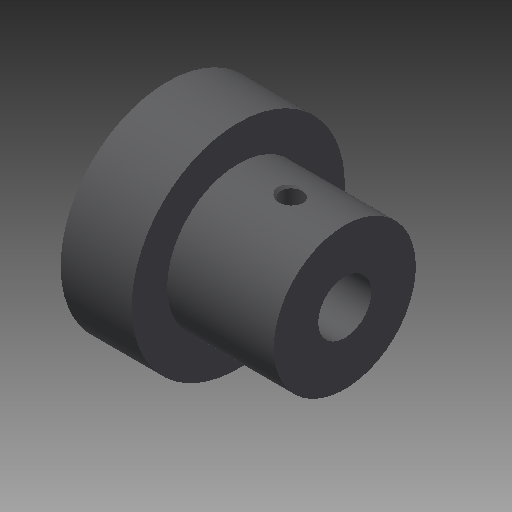
# Autodesk Inventor part: UMHSL30_c
Saved by Autodesk Inventor 2019 (Build 230136000, 136)
## iProperties
Category: PARTsolutions
Company: MISUMI
Created: 2015-12-01
Part Number: UMHSL30_c
Catalog Web Link: www.cadenas.de
Description: UMHSH, UMHS, UMHSL ,UMHAH, UMHA, UMHAL_c-Urethane Rollers with Collars
Vendor: MISUMI
Document SubType Name: Modeling
Designer: psAdmin
Manufacturer: MISUMI
Mass: 5.41814 g
Surface Area: 24.8768 cm^2
Volume: 5.41814 cm^3
Density: 1 g/cm^3
Material: Generic
Appearance: PSOLRGB-192-192-192
PSOL_IDENT_0: {$CADENAS_DATA\23d-libs\misumi\metric\53_rollers\umhsh\umhsh_c.prj},201 {VTYP=3D},{NB=UMHSL30_c},{LI
PSOL_IDENT_1: NA=UMHSL30},{NN=UMHSH, UMHS, UMHSL ,UMHAH, UMHA, UMHAL_c},{DATE=06.11.2015 05:15:16},{GEOMDATE=30.10
PSOL_IDENT_2: .2015 01:04:11},{VERSION=},{LINEID=70},{LINESUBID=-1},{WBVAR=MATC,HARD}  {NB=UMHSL30_c},{LINA=UMHSL3
PSOL_IDENT_3: 0},{KT=DUMMY},{PN=UMHSL30},{TYPE=UMHSL},{MATC=1},{MATU=Urethane (Natural Color)},{HARD=A50},{COLOR=0
PSOL_IDENT_4: .99,1.00,0.74,0.00},{NO=30},{D=30},{DD=6},{D1=16},{D2=24},{D2X=24},{W=8},{L=20},{R=6.0},{M=3}
NN: UMHSH, UMHS, UMHSL ,UMHAH, UMHA, UMHAL_c
NT: Urethane Rollers with Collars
NB: UMHSL30_c
NBSYN: $PN._c
LINA: UMHSL30
PN: UMHSL30
MATC: 304 Stainless Steel
MATU: Urethane (Natural Color)
HARD: Shore A50
D: 30
DD: 6
D1: 16
D2: 24
W: 8
L: 20
R: 6.0
M: 3
SUPPLIER: MISUMI
ARTICLENO: UMHSL30_c
BOMINFO: UMHSL30
CREATOR: CADENAS GmbH
Title: UMHSL30
Author: Cadenas PARTsolutions
Comments: Urethane Rollers with Collars
Autodesk Inventor part; units mm, degrees
sketch "Sketch_2" plane through (0, 0, 0) normal (0, 0, 1) x (1, 0, 0)
  line L0 (12, 0) -> (-8, 0)
  line L1 (-8, 12) -> (-8, 3)
  line L2 (-8, 3) -> (12, 3)
  line L3 (12, 3) -> (12, 8)
  line L4 (12, 8) -> (0, 8)
  line L5 (0, 8) -> (0, 12)
  line L6 (0, 12) -> (-8, 12)
  constraints: 14 end point
revolve "Revolution1" add sketch "Sketch_2" angle 360 about axis through (12, 0, 0) along (1, 0, 0)
sketch "Sketch_4" plane through (0, 0, 0) normal (0, 0, 1) x (1, 0, 0)
  line L0 (6, 0) -> (6, 8)
  line L1 (6, 8) -> (7.5, 8)
  line L2 (7.5, 8) -> (7.2295, 7.7295)
  line L3 (7.2295, 7.7295) -> (7.2295, 0)
  line L4 (7.2295, 0) -> (6, 0)
  line L5 (6, 0) -> (6, 8)
  constraints: 12 end point
revolve "Revolution2" cut sketch "Sketch_4" angle 360 about axis through (6, 0, 0) along (0, -1, 0)
sketch "Sketch_5" plane through (0, 0, 0) normal (0, 1, 0) x (-1, 0, 0)
  line L0 (-6, 0) -> (-6, -8)
  line L1 (-6, -8) -> (-7.5, -8)
  line L2 (-7.5, -8) -> (-7.2295, -7.7295)
  line L3 (-7.2295, -7.7295) -> (-7.2295, 0)
  line L4 (-7.2295, 0) -> (-6, 0)
  line L5 (-6, 0) -> (-6, -8)
  constraints: 12 end point
revolve "Revolution3" cut sketch "Sketch_5" angle 360 about axis through (6, 0, 0) along (0, 0, 1)
thread "Thread1" size "M3x0.5" class "6H" standard "ISO Metric profile" length 4.7295
ref_plane "c_k_XY" through (-4, 0, 0) normal (1, 0, 0) x (0, 0, -1)
ref_plane "c_k_YZ" through (-4, 0, 0) normal (0, 0, -1) x (0, 1, 0)
ref_plane "c_k_ZX" through (-4, 0, 0) normal (0, 1, 0) x (1, 0, 0)
body "Solid1"
